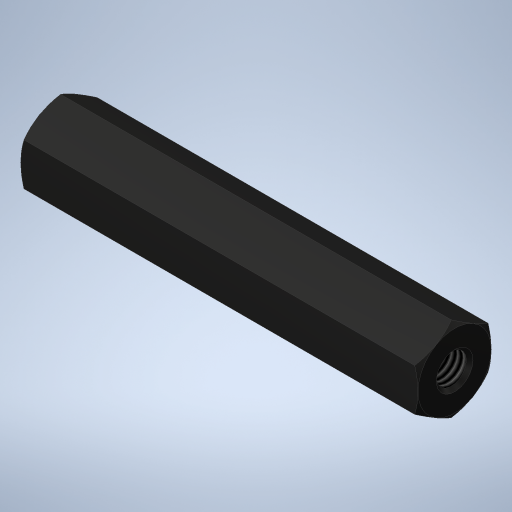
# Autodesk Inventor part: ABLSBF6-32.5-M3-N3
Saved by Autodesk Inventor 2024.2 (Build 282272000, 272)
## iProperties
Created: 2024-04-10
Part Number: ABLSBF6-32.5-M3-N3
Material: Aluminum 2014-T4
Catalog Web Link: www.cadenas.de
Description: NLSBF, LSBF, PLSBF, BLSBF, SLSBF, ALSBF, ABLSBF-Hex Posts - Both Ends Tapped - L Dimension, Thread Dia. Configurable -
Vendor: MISUMI
Document SubType Name: Modeling
Designer: psAdmin
Manufacturer: MISUMI
Mass: 2.60732 g
Surface Area: 8.62228 cm^2
Volume: 0.931186 cm^3
Density: 2.8 g/cm^3
Appearance: Glossy - Black
Category: PARTsolutions
Company: MISUMI
PSOL_IDENT_0: {$CADENAS_DATA/23d-libs/misumi/metric/19_posts_stands/plsbf.prj},255 {VTYP=3D},{NB=ABLSBF6-32.5-M3-N
PSOL_IDENT_1: 3},{LINA=ABLSBF6-32.5-M3-N3},{NN=NLSBF, LSBF, PLSBF, BLSBF, SLSBF, ALSBF, ABLSBF},{DATE=29.05.2023 0
PSOL_IDENT_2: 6:16:11},{GEOMDATE=15.10.2021 09:43:14},{VERSION=},{LINEID=230},{WBVAR=MAT,ST,M,N,ALT1,L,ALT4,ALT2,A
PSOL_IDENT_3: LT3},{WBNUMERIC=M,N,L}  {NB=ABLSBF6-32.5-M3-N3},{LINA=ABLSBF6-32.5-M3-N3},{KT=DUMMY},{PN=ABLSBF6-32.
PSOL_IDENT_4: 5-M3-N3},{TYPE=ABLSBF},{MAT=A2011},{MATALG= 'LCS','Low Carbon Steel','304','SUS304','A2011','A2011-T
PSOL_IDENT_5: 8 Aluminum Alloy' },{ST=BA},{STALG= 'CA','Clear Anodizing','BA','Black Anodizing'},{B=6},{M=3},{MALG=
PSOL_IDENT_6: [3,4]},{N=3},{NALG=[3,4]},{ALT1=},{L=32.5},{LALG=[15:100/0.5]},{LMIN=15},{LMIN1=12},{LMIN1ALG=12},{L
PSOL_IDENT_7: MIN2=15.000},{C=6.9},{ALT4=},{ALT4ALG= '','Not applicable' },{ALT4PN=},{ALT2=},{ALT2ALG='','w/o MD (
PSOL_IDENT_8: Left End Change The Effective Tap Depth)','MD','with MD (Left End Change The Effective Tap Depth)'},
PSOL_IDENT_9: {ALT2PN=},{ALT3=},{ALT3ALG='','w/o ND (Right End Change The Effective Tap Depth)','ND','with ND (Rig
PSOL_IDENT_10: ht End Change The Effective Tap Depth)'},{ALT3PN=},{MAV=3},{MPITCH=0.5},{NPITCH=0.5},{NDEPT=9},{MDEP
PSOL_IDENT_11: T=9},{M3D=6},{N3D=6}
NB: ABLSBF6-32.5-M3-N3
NN: NLSBF, LSBF, PLSBF, BLSBF, SLSBF, ALSBF, ABLSBF
NT: Hex Posts - Both Ends Tapped - L Dimension, Thread Dia. Configurable -
NBSYN: $PN.
LINA: ABLSBF6-32.5-M3-N3
CATALOG: Misumi
PN: ABLSBF6-32.5-M3-N3
MAT: A2011-T8 Aluminum Alloy
ST: Black Anodizing
B: 6
M: 3
N: 3
ALT1: w/o LKC (L Dimension Tolerance)
L: 32.5
C: 6.9
ALT4: Not applicable
ALT2: w/o MD (Left End Change The Effective Tap Depth)
ALT3: w/o ND (Right End Change The Effective Tap Depth)
SUPPLIER: MISUMI
ARTICLENO: ABLSBF6-32.5-M3-N3
BOMINFO: ABLSBF6-32.5-M3-N3
CREATOR: CADENAS GmbH
Title: ABLSBF6-32.5-M3-N3
Author: Cadenas PARTsolutions
Comments: Hex Posts - Both Ends Tapped - L Dimension, Thread Dia. Configurable -
Autodesk Inventor part; units mm, degrees
sketch "Sketch_1" plane through (0, 0, 0) normal (0, 0, 1) x (1, 0, 0)
  line L0 (32.5, 0) -> (0, 0)
  line L1 (0, 0) -> (0, 3)
  line L2 (0, 3) -> (0.5485, 3.95)
  line L3 (0.5485, 3.95) -> (31.9515, 3.95)
  line L4 (31.9515, 3.95) -> (32.5, 3)
  line L5 (32.5, 3) -> (32.5, 0)
  line L6 (32.5, 0) -> (0, 0)
  constraints: 14 end point
revolve "Revolution1" add sketch "Sketch_1" angle 360 about axis through (32.5, 0, 0) along (1, 0, 0)
sketch "Sketch_2" plane through (0, 0, 0) normal (1, 0, 0) x (0, 1, 0)
  line L0 (6, 6) -> (-6, 6)
  line L1 (-6, 6) -> (-6, -6)
  line L2 (-6, -6) -> (6, -6)
  line L3 (6, -6) -> (6, 6)
  line L4 (-1.7321, 3) -> (-3.4641, 0)
  line L5 (-3.4641, 0) -> (-1.7321, -3)
  line L6 (-1.7321, -3) -> (1.7321, -3)
  line L7 (1.7321, -3) -> (3.4641, 0)
  line L8 (3.4641, 0) -> (1.7321, 3)
  line L9 (1.7321, 3) -> (-1.7321, 3)
  constraints: 20 end point
extrude "Extrusion1" cut sketch "Sketch_2" along normal blind 32.5
sketch "Sketch3" plane through (0, 0, 0) normal (-1, 0, 0) x (0, 0, 1)
  point P0 (0, 0)
hole "Hole1" at (0, 0, 0) direction (1, 0, 0) diameter 2.459 depth 8.2901 tip angle 120 countersink diameter 3 countersink angle 90 thread size "M3x0.5" class "6H" standard "ISO Metric profile"
sketch "Sketch4" plane through (32.5, 0, 0) normal (1, 0, 0) x (0, 0, -1)
  point P0 (0, 0)
hole "Hole2" at (32.5, 0, 0) direction (-1, 0, 0) diameter 2.459 depth 8.2901 tip angle 120 countersink diameter 3 countersink angle 90 thread size "M3x0.5" class "6H" standard "ISO Metric profile"
ref_plane "C3_XY" through (32.5, 0, 0) normal (-1, 0, 0) x (0, 0, -1)
ref_plane "C3_YZ" through (32.5, 0, 0) normal (0, 0, -1) x (0, -1, 0)
ref_plane "C3_ZX" through (32.5, 0, 0) normal (0, -1, 0) x (-1, 0, 0)
body "Solid1"
